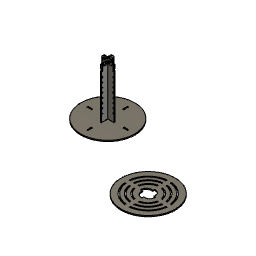
PressurePotRackRotate v5 (Autodesk Fusion 360 design; units mm, degrees)
Autodesk Fusion 360 part; units mm, degrees
(part 1 of 3)
sketch "Sketch1" plane through (0, 0, 0) normal (0, 1, 0) x (1, 0, 0)
  circle A0 centre (0, 0) radius 152.4
  line L0 (0, 0) -> (0, 101.6) construction
  line L1 (0, 0) -> (0, -101.6) construction
  line L2 (0, 0) -> (101.6, 0) construction
  line L3 (0, 0) -> (-101.6, 0) construction
  line L4 (2.9845, 88.9) -> (-2.9845, 88.9)
  line L5 (-2.9845, 88.9) -> (-2.9845, 114.3)
  line L6 (-2.9845, 114.3) -> (2.9845, 114.3)
  line L7 (2.9845, 114.3) -> (2.9845, 88.9)
  line L8 (2.9845, 88.9) -> (-2.9845, 114.3) construction
  line L9 (-2.9845, 88.9) -> (2.9845, 114.3) construction
  line L10 (2.9845, -114.3) -> (-2.9845, -114.3)
  line L11 (-2.9845, -114.3) -> (-2.9845, -88.9)
  line L12 (-2.9845, -88.9) -> (2.9845, -88.9)
  line L13 (2.9845, -88.9) -> (2.9845, -114.3)
  line L14 (2.9845, -114.3) -> (-2.9845, -88.9) construction
  line L15 (-2.9845, -114.3) -> (2.9845, -88.9) construction
  line L16 (114.3, -2.9845) -> (88.9, -2.9845)
  line L17 (88.9, -2.9845) -> (88.9, 2.9845)
  line L18 (88.9, 2.9845) -> (114.3, 2.9845)
  line L19 (114.3, 2.9845) -> (114.3, -2.9845)
  line L20 (114.3, -2.9845) -> (88.9, 2.9845) construction
  line L21 (88.9, -2.9845) -> (114.3, 2.9845) construction
  line L22 (-88.9, -2.9845) -> (-114.3, -2.9845)
  line L23 (-114.3, -2.9845) -> (-114.3, 2.9845)
  line L24 (-114.3, 2.9845) -> (-88.9, 2.9845)
  line L25 (-88.9, 2.9845) -> (-88.9, -2.9845)
  line L26 (-88.9, -2.9845) -> (-114.3, 2.9845) construction
  line L27 (-114.3, -2.9845) -> (-88.9, 2.9845) construction
  line L28 (2.9845, -38.1) -> (-2.9845, -38.1)
  line L29 (-2.9845, -38.1) -> (-2.9845, 38.1)
  line L30 (-2.9845, 38.1) -> (2.9845, 38.1)
  line L31 (2.9845, 38.1) -> (2.9845, -38.1)
  line L32 (2.9845, -38.1) -> (-2.9845, 38.1) construction
  line L33 (-2.9845, -38.1) -> (2.9845, 38.1) construction
  line L34 (38.1, -2.9845) -> (-38.1, -2.9845)
  line L35 (-38.1, -2.9845) -> (-38.1, 2.9845)
  line L36 (-38.1, 2.9845) -> (38.1, 2.9845)
  line L37 (38.1, 2.9845) -> (38.1, -2.9845)
  line L38 (38.1, -2.9845) -> (-38.1, 2.9845) construction
  line L39 (-38.1, -2.9845) -> (38.1, 2.9845) construction
  point P0 (0, 101.6)
  point P1 (0, -101.6)
  point P2 (101.6, 0)
  point P3 (-101.6, 0)
  dimension "d1" = 304.8
  dimension "d2" = 101.6
  dimension "d3" = 101.6
  dimension "d4" = 101.6
  dimension "d5" = 101.6
  dimension "d6" = 5.969
  dimension "d7" = 25.4
  dimension "d8" = 5.969
  dimension "d9" = 25.4
  dimension "d10" = 25.4
  dimension "d11" = 5.969
  dimension "d12" = 25.4
  dimension "d13" = 5.969
  dimension "d14" = 5.969
  dimension "d15" = 76.2
  dimension "d27" = 76.2
  dimension "d28" = 5.969
  constraint coincident A0.centre L0.start
  constraint vertical L0
  constraint parallel L0 L1
  constraint perpendicular L1 L2
  constraint perpendicular L0 L3
  constraint horizontal L4
  constraint perpendicular L4 L5
  constraint parallel L4 L6
  constraint parallel L5 L7
  constraint coincident L8 P0
  constraint coincident L9 P0
  constraint coincident P0 L0.end
  constraint horizontal L10
  constraint perpendicular L10 L11
  constraint parallel L10 L12
  constraint parallel L11 L13
  constraint coincident L14 P1
  constraint coincident L15 P1
  constraint coincident P1 L1.end
  constraint horizontal L16
  constraint perpendicular L16 L17
  constraint parallel L16 L18
  constraint parallel L17 L19
  constraint coincident L20 P2
  constraint coincident L21 P2
  constraint coincident P2 L2.end
  constraint horizontal L22
  constraint perpendicular L22 L23
  constraint parallel L22 L24
  constraint parallel L23 L25
  constraint coincident L26 P3
  constraint coincident L27 P3
  constraint coincident P3 L3.end
  constraint horizontal L28
  constraint perpendicular L28 L29
  constraint parallel L28 L30
  constraint parallel L29 L31
  constraint coincident L32 A0.centre
  constraint coincident L33 A0.centre
  constraint horizontal L34
  constraint perpendicular L34 L35
  constraint parallel L34 L36
  constraint parallel L35 L37
  constraint coincident L38 A0.centre
  constraint coincident L39 A0.centre
  measures "d1" diameter of A0
  measures "d2" distance of A0.centre P0
  measures "d3" distance of A0.centre P1
  measures "d4" distance of A0.centre P2
  measures "d5" distance of A0.centre P3
  measures "d6" distance of L5.end L6.end
  measures "d7" distance of L4.end L5.end
  measures "d8" distance of L11.end L12.end
  measures "d9" distance of L10.end L11.end
  measures "d10" distance of L17.end L18.end
  measures "d11" distance of L16.end L17.end
  measures "d12" distance of L23.end L24.end
  measures "d13" distance of L22.end L23.end
  measures "d14" distance of L29.end L30.end
  measures "d15" distance of L28.end L29.end
  measures "d27" distance of L35.end L36.end
  measures "d28" distance of L34.end L35.end
extrude "Extrude1" add sketch "Sketch1" along normal blind 5.969 contours A0 | L31 L34 L36 L37 | L29 L34 L35 L36 makes body 1 in component "Component"
sketch "Sketch2" plane through (0, 0, 0) normal (0, -1, 0) x (1, 0, 0)
  line L0 (2.9845, 88.9) -> (-2.9845, 88.9)
  line L1 (-2.9845, 88.9) -> (-2.9845, 114.3)
  line L2 (-2.9845, 114.3) -> (2.9845, 114.3)
  line L3 (2.9845, 114.3) -> (2.9845, 88.9)
  line L4 (114.3, -2.9845) -> (88.9, -2.9845)
  line L5 (88.9, -2.9845) -> (88.9, 2.9845)
  line L6 (88.9, 2.9845) -> (114.3, 2.9845)
  line L7 (114.3, 2.9845) -> (114.3, -2.9845)
  line L8 (-88.9, -2.9845) -> (-114.3, -2.9845)
  line L9 (-114.3, -2.9845) -> (-114.3, 2.9845)
  line L10 (-114.3, 2.9845) -> (-88.9, 2.9845)
  line L11 (-88.9, 2.9845) -> (-88.9, -2.9845)
  line L12 (2.9845, -114.3) -> (-2.9845, -114.3)
  line L13 (-2.9845, -114.3) -> (-2.9845, -88.9)
  line L14 (-2.9845, -88.9) -> (2.9845, -88.9)
  line L15 (2.9845, -88.9) -> (2.9845, -114.3)
  line L16 (2.9845, -38.1) -> (-2.9845, -38.1)
  line L17 (-2.9845, -38.1) -> (-2.9845, 38.1)
  line L18 (-2.9845, 38.1) -> (2.9845, 38.1)
  line L19 (2.9845, 38.1) -> (2.9845, -38.1)
  circle A0 centre (0, 0) radius 152.4
  line L20 (-114.3, 2.9845) -> (114.3, 2.9845)
  line L21 (114.3, 2.9845) -> (114.3, -2.9845)
  line L22 (114.3, -2.9845) -> (-114.3, -2.9845)
  line L23 (-114.3, -2.9845) -> (-114.3, 2.9845)
  constraint horizontal L20
  constraint vertical L21
  constraint horizontal L22
  constraint vertical L23
  constraint coincident L4.start L7.end
  constraint coincident L9.end L10.start
extrude "Extrude1'" add sketch "Sketch2" along normal blind 19.05 separate body contours L4 L5 L6 L7 L20 L21 L22 | L5 L19 L20 L22 | L17 L19 L20 L22 | L11 L17 L20 L22 | L8 L9 L10 L11 L20 L22 L23 makes body 2
extrude "Extrude2" add sketch "Sketch2" against normal blind 5.969 contours L4 L5 L6 L7 L20 L21 L22 bodies 2
extrude "Extrude3" add sketch "Sketch2" against normal blind 5.969 contours L8 L9 L10 L11 L20 L22 L23 bodies 2
sketch "Sketch3" plane through (0, -19.05, 0) normal (0, -1, 0) x (1, 0, 0)
  line L0 (-114.3, -2.9845) -> (114.3, -2.9845)
  line L1 (114.3, -2.9845) -> (114.3, 2.9845)
  line L2 (114.3, 2.9845) -> (-114.3, 2.9845)
  line L3 (-114.3, 2.9845) -> (-114.3, -2.9845)
  line L4 (2.9845, -2.9845) -> (-2.9845, -2.9845)
  line L5 (-2.9845, -2.9845) -> (-2.9845, 2.9845)
  line L6 (-2.9845, 2.9845) -> (2.9845, 2.9845)
  line L7 (2.9845, 2.9845) -> (2.9845, -2.9845)
  line L8 (2.9845, -2.9845) -> (-2.9845, 2.9845) construction
  line L9 (-2.9845, -2.9845) -> (2.9845, 2.9845) construction
  dimension "d24" = 5.969
  constraint horizontal L4
  constraint perpendicular L4 L5
  constraint parallel L4 L6
  constraint parallel L5 L7
  constraint coincident L8 origin
  constraint coincident L9 origin
  measures "d24" distance of L5.end L6.end
extrude "Extrude4" cut sketch "Sketch3" against normal blind 9.525 contours L0 L2 L4 L5 L6 L7 bodies 2
copy_body "Body->Comp1" bodies 2 removing the originals makes body 3 in component "Component'"
extrude "Extrude2'" cut sketch "Sketch1" along normal up to surface (5.969 mm away) contours L31 L34 L36 L37 | L29 L34 L35 L36 bodies 1 in component "Component"
sketch "Sketch4" plane through (0, 0, 0) normal (0, -1, 0) x (1, 0, 0)
  line L0 (-38.1, 2.9845) -> (-2.9845, 2.9845)
  line L1 (-2.9845, 2.9845) -> (-2.9845, 38.1)
  line L2 (-2.9845, 38.1) -> (2.9845, 38.1)
  line L3 (2.9845, 38.1) -> (2.9845, 2.9845)
  line L4 (2.9845, 2.9845) -> (38.1, 2.9845)
  line L5 (38.1, 2.9845) -> (38.1, -2.9845)
  line L6 (38.1, -2.9845) -> (2.9845, -2.9845)
  line L7 (2.9845, -2.9845) -> (2.9845, -38.1)
  line L8 (2.9845, -38.1) -> (-2.9845, -38.1)
  line L9 (-2.9845, -38.1) -> (-2.9845, -2.9845)
  line L10 (-2.9845, -2.9845) -> (-38.1, -2.9845)
  line L11 (-38.1, -2.9845) -> (-38.1, 2.9845)
  line L12 (2.9845, -114.3) -> (-2.9845, -114.3)
  line L13 (-2.9845, -114.3) -> (-2.9845, -88.9)
  line L14 (-2.9845, -88.9) -> (2.9845, -88.9)
  line L15 (2.9845, -88.9) -> (2.9845, -114.3)
  line L16 (-88.9, -2.9845) -> (-114.3, -2.9845)
  line L17 (-114.3, -2.9845) -> (-114.3, 2.9845)
  line L18 (-114.3, 2.9845) -> (-88.9, 2.9845)
  line L19 (-88.9, 2.9845) -> (-88.9, -2.9845)
  line L20 (114.3, -2.9845) -> (88.9, -2.9845)
  line L21 (88.9, -2.9845) -> (88.9, 2.9845)
  line L22 (88.9, 2.9845) -> (114.3, 2.9845)
  line L23 (114.3, 2.9845) -> (114.3, -2.9845)
  line L24 (2.9845, 88.9) -> (-2.9845, 88.9)
  line L25 (-2.9845, 88.9) -> (-2.9845, 114.3)
  line L26 (-2.9845, 114.3) -> (2.9845, 114.3)
  line L27 (2.9845, 114.3) -> (2.9845, 88.9)
  circle A0 centre (0, 0) radius 152.4
  line L28 (2.9845, -114.3) -> (-2.9845, -114.3)
  line L29 (-2.9845, -114.3) -> (-2.9845, 114.3)
  line L30 (-2.9845, 114.3) -> (2.9845, 114.3)
  line L31 (2.9845, 114.3) -> (2.9845, -114.3)
  line L32 (2.9845, -114.3) -> (-2.9845, 114.3) construction
  line L33 (-2.9845, -114.3) -> (2.9845, 114.3) construction
  constraint horizontal L28
  constraint perpendicular L28 L29
  constraint parallel L28 L30
  constraint parallel L29 L31
  constraint coincident L12.start L15.end
  constraint coincident L32 A0.centre
  constraint coincident L33 A0.centre
  constraint coincident A0.centre origin
extrude "Extrude1''" add sketch "Sketch4" along normal blind 19.05 separate body contours L1 L2 L3 L7 L8 L9 L29 L31 | L2 L24 L29 L31 | L24 L25 L26 L27 L29 L30 L31 | L8 L14 L29 L31 | L12 L13 L14 L15 L28 L29 L31 makes body 4 in component "Component''"
sketch "Sketch5" plane through (0, 0, 0) normal (0, 1, 0) x (-1, 0, 0)
  line L0 (2.9845, 114.3) -> (-2.9845, 114.3)
  line L1 (-2.9845, 114.3) -> (-2.9845, -114.3)
  line L2 (-2.9845, -114.3) -> (2.9845, -114.3)
  line L3 (2.9845, -114.3) -> (2.9845, 114.3)
  line L4 (-2.9845, 2.9845) -> (2.9845, 2.9845)
  line L5 (2.9845, 2.9845) -> (2.9845, -2.9845)
  line L6 (2.9845, -2.9845) -> (-2.9845, -2.9845)
  line L7 (-2.9845, -2.9845) -> (-2.9845, 2.9845)
  line L8 (-2.9845, 2.9845) -> (2.9845, -2.9845) construction
  line L9 (2.9845, 2.9845) -> (-2.9845, -2.9845) construction
  line L10 (-2.9845, -114.3) -> (2.9845, -114.3)
  line L11 (2.9845, -114.3) -> (2.9845, -88.9)
  line L12 (2.9845, -88.9) -> (-2.9845, -88.9)
  line L13 (-2.9845, -88.9) -> (-2.9845, -114.3)
  line L14 (-2.9845, 114.3) -> (2.9845, 114.3)
  line L15 (2.9845, 114.3) -> (2.9845, 88.9)
  line L16 (2.9845, 88.9) -> (-2.9845, 88.9)
  line L17 (-2.9845, 88.9) -> (-2.9845, 114.3)
  dimension "d33" = 5.969
  dimension "d34" = 25.4
  dimension "d35" = 25.4
  constraint horizontal L4
  constraint perpendicular L4 L5
  constraint parallel L4 L6
  constraint parallel L5 L7
  constraint coincident L8 origin
  constraint coincident L9 origin
  constraint horizontal L10
  constraint vertical L11
  constraint horizontal L12
  constraint vertical L13
  constraint coincident L1.end L2.start
  constraint horizontal L14
  constraint vertical L15
  constraint horizontal L16
  constraint vertical L17
  constraint coincident L0.end L1.start
  measures "d33" distance of L4.end L5.end
  measures "d34" distance of L1.end L12.end
  measures "d35" distance of L0.end L16.end
extrude "Extrude2''" cut sketch "Sketch5" against normal blind 9.525 contours L1 L3 L4 L5 L6 L7 bodies 4 in component "Component''"
extrude "Extrude3'" add sketch "Sketch5" along normal blind 5.969 contours L0 L1 L3 L14 L15 L16 L17 bodies 4 in component "Component''"
extrude "Extrude4'" add sketch "Sketch5" along normal blind 5.969 contours L1 L2 L3 L10 L11 L12 L13 bodies 4 in component "Component''"
sketch "Sketch6" plane through (0, 0, 0) normal (0, 1, 0) x (-1, 0, 0)
  line L0 (88.9, -2.9845) -> (88.9, 2.9845)
  line L1 (88.9, 2.9845) -> (-88.9, 2.9845)
  line L2 (-88.9, 2.9845) -> (-88.9, -2.9845)
  line L3 (-88.9, -2.9845) -> (88.9, -2.9845)
  line L4 (-38.1, 2.9845) -> (38.1, 2.9845)
  line L5 (38.1, 2.9845) -> (38.1, -2.9845)
  line L6 (38.1, -2.9845) -> (-38.1, -2.9845)
  line L7 (-38.1, -2.9845) -> (-38.1, 2.9845)
  line L8 (-38.1, 2.9845) -> (38.1, -2.9845) construction
  line L9 (38.1, 2.9845) -> (-38.1, -2.9845) construction
  dimension "d42" = 76.2
  constraint horizontal L4
  constraint perpendicular L4 L5
  constraint parallel L4 L6
  constraint parallel L5 L7
  constraint coincident L8 origin
  constraint coincident L9 origin
  measures "d42" distance of L5.end L6.end
extrude "Extrude1'''" add sketch "Sketch6" along normal blind 304.8 contours L1 L3 L4 L5 L6 L7 bodies 3 in component "Component'"
sketch "Sketch7" plane through (0, 0, 0) normal (0, 1, 0) x (-1, 0, 0)
  line L0 (2.9845, 88.9) -> (-2.9845, 88.9)
  line L1 (-2.9845, 88.9) -> (-2.9845, 2.9845)
  line L2 (-2.9845, 2.9845) -> (2.9845, 2.9845)
  line L3 (2.9845, 2.9845) -> (2.9845, 88.9)
  line L4 (2.9845, 2.9845) -> (-2.9845, 2.9845)
  line L5 (-2.9845, 2.9845) -> (-2.9845, 38.1)
  line L6 (-2.9845, 38.1) -> (2.9845, 38.1)
  line L7 (2.9845, 38.1) -> (2.9845, 2.9845)
  dimension "d45" = 35.1155
  constraint horizontal L4
  constraint vertical L5
  constraint horizontal L6
  constraint vertical L7
  constraint coincident L2.end L3.start
  measures "d45" distance of L2.end L6.end
extrude "Extrude5" add sketch "Sketch7" along normal blind 304.8 contours L1 L2 L3 L4 L5 L6 L7 bodies 4 in component "Component''"
sketch "Sketch8" plane through (0, 0, 0) normal (0, 1, 0) x (-1, 0, 0)
  line L0 (-2.9845, -88.9) -> (2.9845, -88.9)
  line L1 (2.9845, -88.9) -> (2.9845, -2.9845)
  line L2 (2.9845, -2.9845) -> (-2.9845, -2.9845)
  line L3 (-2.9845, -2.9845) -> (-2.9845, -88.9)
  line L4 (2.9845, -2.9845) -> (-2.9845, -2.9845)
  line L5 (-2.9845, -2.9845) -> (-2.9845, -38.1)
  line L6 (-2.9845, -38.1) -> (2.9845, -38.1)
  line L7 (2.9845, -38.1) -> (2.9845, -2.9845)
  dimension "d48" = 35.1155
  constraint horizontal L4
  constraint vertical L5
  constraint horizontal L6
  constraint vertical L7
  constraint coincident L1.end L2.start
  measures "d48" distance of L1.end L6.end
extrude "Extrude6" add sketch "Sketch8" along normal blind 304.8 contours L1 L2 L3 L4 L5 L6 L7 bodies 4 in component "Component''"
fillet "Fillet1" radius 12.7 2 edges at (114.3, -19.05, 0) (-114.3, -19.05, 0) on bodies 3 in component "Component'"
fillet "Fillet1'" radius 12.7 2 edges at (0, -19.05, 114.3) (0, -19.05, -114.3) on bodies 4 in component "Component''"
sketch "Sketch9" plane through (-38.1, 0, 0) normal (-1, 0, 0) x (0, 0, 1)
  line L0 (-2.9845, 0) -> (2.9845, 0)
  line L1 (2.9845, 0) -> (2.9845, 304.8)
  line L2 (2.9845, 304.8) -> (-2.9845, 304.8)
  line L3 (-2.9845, 304.8) -> (-2.9845, 0)
  line L4 (-2.9845, 304.8) -> (2.9845, 304.8)
  line L5 (2.9845, 304.8) -> (2.9845, 254)
  line L6 (2.9845, 254) -> (-2.9845, 254)
  line L7 (-2.9845, 254) -> (-2.9845, 304.8)
  dimension "d55" = 50.8
  constraint horizontal L4
  constraint vertical L5
  constraint horizontal L6
  constraint vertical L7
  constraint coincident L2.end L3.start
  measures "d55" distance of L2.end L6.end
extrude "Extrude2'''" cut sketch "Sketch9" against normal blind 6.35 contours L1 L2 L3 L4 L5 L6 L7 bodies 3 in component "Component'"
sketch "Sketch10" plane through (0, 0, -38.1) normal (0, 0, -1) x (-1, 0, 0)
  line L0 (-2.9845, 0) -> (2.9845, 0)
  line L1 (2.9845, 0) -> (2.9845, 304.8)
  line L2 (2.9845, 304.8) -> (-2.9845, 304.8)
  line L3 (-2.9845, 304.8) -> (-2.9845, 0)
  line L4 (-2.9845, 304.8) -> (2.9845, 304.8)
  line L5 (2.9845, 304.8) -> (2.9845, 254)
  line L6 (2.9845, 254) -> (-2.9845, 254)
  line L7 (-2.9845, 254) -> (-2.9845, 304.8)
  dimension "d58" = 50.8
  constraint horizontal L4
  constraint vertical L5
  constraint horizontal L6
  constraint vertical L7
  constraint coincident L2.end L3.start
  measures "d58" distance of L2.end L6.end
extrude "Extrude7" cut sketch "Sketch10" against normal blind 6.35 contours L1 L2 L3 L4 L5 L6 L7 bodies 4 in component "Component''"
sketch "Sketch11" plane through (38.1, 0, 0) normal (1, 0, 0) x (0, 0, -1)
  line L0 (-2.9845, 0) -> (2.9845, 0)
  line L1 (2.9845, 0) -> (2.9845, 304.8)
  line L2 (2.9845, 304.8) -> (-2.9845, 304.8)
  line L3 (-2.9845, 304.8) -> (-2.9845, 0)
  line L4 (-2.9845, 304.8) -> (2.9845, 304.8)
  line L5 (2.9845, 304.8) -> (2.9845, 254)
  line L6 (2.9845, 254) -> (-2.9845, 254)
  line L7 (-2.9845, 254) -> (-2.9845, 304.8)
  dimension "d61" = 5.969
  dimension "d62" = 50.8
  constraint horizontal L4
  constraint vertical L5
  constraint horizontal L6
  constraint vertical L7
  constraint coincident L2.end L3.start
  measures "d61" distance of L2.end L1.end
  measures "d62" distance of L2.end L6.end
extrude "Extrude3''" cut sketch "Sketch11" against normal blind 6.35 contours L1 L2 L3 L4 L5 L6 L7 bodies 3 in component "Component'"
sketch "Sketch12" plane through (0, 0, 38.1) normal (0, 0, 1) x (1, 0, 0)
  line L0 (-2.9845, 0) -> (2.9845, 0)
  line L1 (2.9845, 0) -> (2.9845, 304.8)
  line L2 (2.9845, 304.8) -> (-2.9845, 304.8)
  line L3 (-2.9845, 304.8) -> (-2.9845, 0)
  line L4 (-2.9845, 304.8) -> (2.9845, 304.8)
  line L5 (2.9845, 304.8) -> (2.9845, 254)
  line L6 (2.9845, 254) -> (-2.9845, 254)
  line L7 (-2.9845, 254) -> (-2.9845, 304.8)
  dimension "d65" = 50.8
  constraint horizontal L4
  constraint vertical L5
  constraint horizontal L6
  constraint vertical L7
  constraint coincident L2.end L3.start
  measures "d65" distance of L2.end L6.end
extrude "Extrude8" cut sketch "Sketch12" against normal blind 6.35 contours L1 L2 L3 L4 L5 L6 L7 bodies 4 in component "Component''"
fillet "Fillet2" radius 12.7 2 edges at (31.75, 304.8, 0) (-31.75, 304.8, 0) on bodies 3 in component "Component'"
fillet "Fillet2'" radius 12.7 2 edges at (0, 304.8, -31.75) (0, 304.8, 31.75) on bodies 4 in component "Component''"
sketch "Sketch13" plane through (-2.9845, 0, 0) normal (-1, 0, 0) x (0, 0, 1)
  arc A0 (31.75, 292.1) -> (19.05, 304.8) centre (19.05, 292.1) ccw
  line L0 (19.05, 304.8) -> (2.9845, 304.8)
  line L1 (2.9845, 304.8) -> (2.9845, -9.525)
  line L2 (2.9845, -9.525) -> (-2.9845, -9.525)
  line L3 (-2.9845, -9.525) -> (-2.9845, 304.8)
  line L4 (-2.9845, 304.8) -> (-19.05, 304.8)
  arc A1 (-19.05, 304.8) -> (-31.75, 292.1) centre (-19.05, 292.1) ccw
  line L5 (-31.75, 292.1) -> (-31.75, 254)
  line L6 (-31.75, 254) -> (-38.1, 254)
  line L7 (-38.1, 254) -> (-38.1, 0)
  line L8 (-38.1, 0) -> (-88.9, 0)
  line L9 (-88.9, 0) -> (-88.9, 5.969)
  line L10 (-88.9, 5.969) -> (-114.3, 5.969)
  line L11 (-114.3, 5.969) -> (-114.3, -6.35)
  arc A2 (-114.3, -6.35) -> (-101.6, -19.05) centre (-101.6, -6.35) ccw
  line L12 (-101.6, -19.05) -> (101.6, -19.05)
  arc A3 (101.6, -19.05) -> (114.3, -6.35) centre (101.6, -6.35) ccw
  line L13 (114.3, -6.35) -> (114.3, 5.969)
  line L14 (114.3, 5.969) -> (88.9, 5.969)
  line L15 (88.9, 5.969) -> (88.9, 0)
  line L16 (88.9, 0) -> (38.1, 0)
  line L17 (38.1, 0) -> (38.1, 254)
  line L18 (38.1, 254) -> (31.75, 254)
  line L19 (31.75, 254) -> (31.75, 292.1)
  line L20 (2.9845, 304.8) -> (17.3736, 304.8) construction
  line L21 (17.3736, 304.8) -> (17.3736, 285.75) construction
  line L22 (-2.9845, 304.8) -> (-17.3736, 304.8) construction
  line L23 (-17.3736, 304.8) -> (-17.3736, 285.75) construction
  circle A4 centre (17.3736, 285.75) radius 11.1125
  circle A5 centre (-17.3736, 285.75) radius 11.1125
  dimension "d72" = 14.3891
  dimension "d73" = 19.05
  dimension "d74" = 14.3891
  dimension "d75" = 19.05
  dimension "d76" = 22.225
  dimension "d77" = 22.225
  constraint coincident L0.end L1.start
  constraint perpendicular L1 L20
  constraint perpendicular L20 L21
  constraint coincident L3.end L4.start
  constraint perpendicular L3 L22
  constraint perpendicular L22 L23
  constraint coincident L21.end A4.centre
  constraint coincident L23.end A5.centre
  measures "d72" distance of L0.end L20.end
  measures "d73" distance of L20.end L21.end
  measures "d74" distance of L3.end L22.end
  measures "d75" distance of L22.end L23.end
  measures "d76" diameter of A4
  measures "d77" diameter of A5
extrude "Extrude9" cut sketch "Sketch13" against normal up to surface (5.969 mm away) contours A4 bodies 4 in component "Component''"
extrude "Extrude10" cut sketch "Sketch13" against normal up to surface (5.969 mm away) contours A5 bodies 4 in component "Component''"
sketch "Sketch14" plane through (0, 0, -2.9845) normal (0, 0, -1) x (-1, 0, 0)
  arc A0 (31.75, 292.1) -> (19.05, 304.8) centre (19.05, 292.1) ccw
  line L0 (19.05, 304.8) -> (-19.05, 304.8)
  arc A1 (-19.05, 304.8) -> (-31.75, 292.1) centre (-19.05, 292.1) ccw
  line L1 (-31.75, 292.1) -> (-31.75, 254)
  line L2 (-31.75, 254) -> (-38.1, 254)
  line L3 (-38.1, 254) -> (-38.1, 0)
  line L4 (-38.1, 0) -> (-88.9, 0)
  line L5 (-88.9, 0) -> (-88.9, 5.969)
  line L6 (-88.9, 5.969) -> (-114.3, 5.969)
  line L7 (-114.3, 5.969) -> (-114.3, -6.35)
  arc A2 (-114.3, -6.35) -> (-101.6, -19.05) centre (-101.6, -6.35) ccw
  line L8 (-101.6, -19.05) -> (-2.9845, -19.05)
  line L9 (-2.9845, -19.05) -> (-2.9845, -9.525)
  line L10 (-2.9845, -9.525) -> (2.9845, -9.525)
  line L11 (2.9845, -9.525) -> (2.9845, -19.05)
  line L12 (2.9845, -19.05) -> (101.6, -19.05)
  arc A3 (101.6, -19.05) -> (114.3, -6.35) centre (101.6, -6.35) ccw
  line L13 (114.3, -6.35) -> (114.3, 5.969)
  line L14 (114.3, 5.969) -> (88.9, 5.969)
  line L15 (88.9, 5.969) -> (88.9, 0)
  line L16 (88.9, 0) -> (38.1, 0)
  line L17 (38.1, 0) -> (38.1, 254)
  line L18 (38.1, 254) -> (31.75, 254)
  line L19 (31.75, 254) -> (31.75, 292.1)
  line L20 (-31.75, 292.1) -> (-31.75, 285.75) construction
  line L21 (31.75, 292.1) -> (31.75, 285.75) construction
  line L22 (-31.75, 285.75) -> (-17.3609, 285.75) construction
  line L23 (31.75, 285.75) -> (17.3609, 285.75) construction
  circle A4 centre (17.3609, 285.75) radius 11.1125
  circle A5 centre (-17.3609, 285.75) radius 11.1125
  dimension "d82" = 6.35
  dimension "d83" = 6.35
  dimension "d84" = 14.3891
  dimension "d85" = 14.3891
  dimension "d86" = 22.225
  dimension "d87" = 22.225
  constraint coincident A1.end L1.start
  constraint perpendicular L0 L20
  constraint coincident A0.start L19.end
  constraint parallel L19 L21
  constraint perpendicular L20 L22
  constraint perpendicular L21 L23
  constraint coincident L23.end A4.centre
  constraint coincident L22.end A5.centre
  measures "d82" distance of A1.end L20.end
  measures "d83" distance of A0.start L21.end
  measures "d84" distance of L20.end L22.end
  measures "d85" distance of L21.end L23.end
  measures "d86" diameter of A4
  measures "d87" diameter of A5
extrude "Extrude4''" cut sketch "Sketch14" against normal up to surface (5.969 mm away) contours A4 | A5 bodies 3 in component "Component'"
sketch "Sketch15" plane through (0, 0, 0) normal (0, 1, 0) x (1, 0, 0)
  circle A0 centre (482.6, -254) radius 152.4
  line L0 (485.5845, -285.75) -> (479.6155, -285.75)
  line L1 (479.6155, -285.75) -> (479.6155, -222.25)
  line L2 (479.6155, -222.25) -> (485.5845, -222.25)
  line L3 (485.5845, -222.25) -> (485.5845, -285.75)
  line L4 (485.5845, -285.75) -> (479.6155, -222.25) construction
  line L5 (479.6155, -285.75) -> (485.5845, -222.25) construction
  line L6 (514.35, -256.9845) -> (450.85, -256.9845)
  line L7 (450.85, -256.9845) -> (450.85, -251.0155)
  line L8 (450.85, -251.0155) -> (514.35, -251.0155)
  line L9 (514.35, -251.0155) -> (514.35, -256.9845)
  line L10 (514.35, -256.9845) -> (450.85, -251.0155) construction
  line L11 (450.85, -256.9845) -> (514.35, -251.0155) construction
  point P0 (482.6, -254)
  point P1 (482.6, -254)
  dimension "d90" = 304.8
  dimension "d91" = 5.969
  dimension "d92" = 63.5
  dimension "d93" = 63.5
  dimension "d94" = 5.969
  constraint horizontal L0
  constraint perpendicular L0 L1
  constraint parallel L0 L2
  constraint parallel L1 L3
  constraint coincident L4 P1
  constraint coincident L5 P1
  constraint coincident P0 A0.centre
  constraint horizontal L6
  constraint perpendicular L6 L7
  constraint parallel L6 L8
  constraint parallel L7 L9
  constraint coincident L10 P1
  constraint coincident L11 P1
  constraint coincident P1 P0
  measures "d90" diameter of A0
  measures "d91" distance of L1.end L2.end
  measures "d92" distance of L0.end L1.end
  measures "d93" distance of L7.end L8.end
  measures "d94" distance of L6.end L7.end
extrude "Extrude5'" add sketch "Sketch15" along normal blind 5.969 separate body makes body 5
sketch "Sketch16" plane through (0, 5.969, 0) normal (0, 1, 0) x (-1, 0, 0)
  line L0 (-485.5845, 251.0155) -> (-514.35, 251.0155)
  line L1 (-514.35, 251.0155) -> (-514.35, 256.9845)
  line L2 (-514.35, 256.9845) -> (-485.5845, 256.9845)
  line L3 (-485.5845, 256.9845) -> (-485.5845, 285.75)
  line L4 (-485.5845, 285.75) -> (-479.6155, 285.75)
  line L5 (-479.6155, 285.75) -> (-479.6155, 256.9845)
  line L6 (-479.6155, 256.9845) -> (-450.85, 256.9845)
  line L7 (-450.85, 256.9845) -> (-450.85, 251.0155)
  line L8 (-450.85, 251.0155) -> (-479.6155, 251.0155)
  line L9 (-479.6155, 251.0155) -> (-479.6155, 222.25)
  line L10 (-479.6155, 222.25) -> (-485.5845, 222.25)
  line L11 (-485.5845, 222.25) -> (-485.5845, 251.0155)
  circle A0 centre (-482.6, 254) radius 152.4
  circle A1 centre (-482.6, 254) radius 63.5
  circle A2 centre (-482.6, 254) radius 69.85
  circle A3 centre (-482.6, 254) radius 88.9
  circle A4 centre (-482.6, 254) radius 95.25
  circle A5 centre (-482.6, 254) radius 114.3
  circle A6 centre (-482.6, 254) radius 120.65
  line L12 (-495.3, 381) -> (-469.9, 381)
  line L13 (-469.9, 381) -> (-469.9, 127)
  line L14 (-469.9, 127) -> (-495.3, 127)
  line L15 (-495.3, 127) -> (-495.3, 381)
  line L16 (-495.3, 381) -> (-469.9, 127) construction
  line L17 (-469.9, 381) -> (-495.3, 127) construction
  line L18 (-609.6, 266.7) -> (-355.6, 266.7)
  line L19 (-355.6, 266.7) -> (-355.6, 241.3)
  line L20 (-355.6, 241.3) -> (-609.6, 241.3)
  line L21 (-609.6, 241.3) -> (-609.6, 266.7)
  line L22 (-609.6, 266.7) -> (-355.6, 241.3) construction
  line L23 (-355.6, 266.7) -> (-609.6, 241.3) construction
  point P0 (-482.6, 254)
  point P1 (-482.6, 254)
  dimension "d98" = 127
  dimension "d99" = 139.7
  dimension "d100" = 177.8
  dimension "d101" = 190.5
  dimension "d102" = 228.6
  dimension "d103" = 241.3
  dimension "d104" = 254
  dimension "d105" = 25.4
  constraint concentric A0 A1
  constraint concentric A1 A2
  constraint concentric A2 A3
  constraint concentric A1 A4
  constraint concentric A3 A5
  constraint concentric A3 A6
  constraint horizontal L12
  constraint perpendicular L12 L13
  constraint parallel L12 L14
  constraint parallel L13 L15
  constraint coincident L16 P1
  constraint coincident L17 P1
  constraint coincident P1 P0
  constraint horizontal L18
  constraint perpendicular L18 L19
  constraint parallel L18 L20
  constraint parallel L19 L21
  constraint coincident L22 P1
  constraint coincident L23 P1
  measures "d98" diameter of A1
  measures "d99" diameter of A2
  measures "d100" diameter of A3
  measures "d101" diameter of A4
  measures "d102" diameter of A5
  measures "d103" diameter of A6
  measures "d104" distance of L19.end L20.end
  measures "d105" distance of L18.end L19.end
extrude "Extrude6'" cut sketch "Sketch16" against normal up to surface (5.969 mm away) contours A1 A2 L15 L20 | A1 A2 L13 L20 | A1 A2 L15 L18 | A3 A4 L15 L20 | A1 A2 L13 L18 | A3 A4 L13 L20 | A3 A4 L15 L18 | A5 A6 L15 L20 | A3 A4 L13 L18 | A5 A6 L13 L20 | A5 A6 L15 L18 | A5 A6 L13 L18 bodies 5
copy_body "Body->Comp2" bodies 5 removing the originals makes body 6 in component "Component'''"
sketch "Sketch17" plane through (0, 5.969, 0) normal (0, 1, 0) x (-1, 0, 0)
  arc A0 (-495.3, 367.5922) -> (-596.1922, 266.7) centre (-482.6, 254) ccw
  line L0 (-596.1922, 266.7) -> (-602.5797, 266.7)
  arc A1 (-495.3, 373.9797) -> (-602.5797, 266.7) centre (-482.6, 254) ccw
  line L1 (-495.3, 373.9797) -> (-495.3, 367.5922)
  arc A2 (-469.9, 166.0118) -> (-394.6118, 241.3) centre (-482.6, 254) ccw
  line L2 (-394.6118, 241.3) -> (-388.2005, 241.3)
  arc A3 (-469.9, 159.6005) -> (-388.2005, 241.3) centre (-482.6, 254) ccw
  line L3 (-469.9, 159.6005) -> (-469.9, 166.0118)
  arc A4 (-420.383, 266.7) -> (-469.9, 316.217) centre (-482.6, 254) ccw
  line L4 (-469.9, 316.217) -> (-469.9, 322.6857)
  arc A5 (-413.9142, 266.7) -> (-469.9, 322.6857) centre (-482.6, 254) ccw
  line L5 (-413.9142, 266.7) -> (-420.383, 266.7)
  arc A6 (-469.9, 191.783) -> (-420.383, 241.3) centre (-482.6, 254) ccw
  line L6 (-420.383, 241.3) -> (-413.9142, 241.3)
  arc A7 (-469.9, 185.3142) -> (-413.9142, 241.3) centre (-482.6, 254) ccw
  line L7 (-469.9, 185.3142) -> (-469.9, 191.783)
  arc A8 (-394.6118, 266.7) -> (-469.9, 341.9882) centre (-482.6, 254) ccw
  line L8 (-469.9, 341.9882) -> (-469.9, 348.3995)
  arc A9 (-388.2005, 266.7) -> (-469.9, 348.3995) centre (-482.6, 254) ccw
  line L9 (-388.2005, 266.7) -> (-394.6118, 266.7)
  arc A10 (-469.9, 140.4077) -> (-369.0077, 241.3) centre (-482.6, 254) ccw
  line L10 (-369.0077, 241.3) -> (-362.6203, 241.3)
  arc A11 (-469.9, 134.0203) -> (-362.6203, 241.3) centre (-482.6, 254) ccw
  line L11 (-469.9, 134.0203) -> (-469.9, 140.4077)
  arc A12 (-369.0077, 266.7) -> (-469.9, 367.5922) centre (-482.6, 254) ccw
  line L12 (-469.9, 367.5922) -> (-469.9, 373.9797)
  arc A13 (-362.6203, 266.7) -> (-469.9, 373.9797) centre (-482.6, 254) ccw
  line L13 (-362.6203, 266.7) -> (-369.0077, 266.7)
  arc A14 (-570.5882, 241.3) -> (-495.3, 166.0118) centre (-482.6, 254) ccw
  line L14 (-495.3, 166.0118) -> (-495.3, 159.6005)
  arc A15 (-576.9995, 241.3) -> (-495.3, 159.6005) centre (-482.6, 254) ccw
  line L15 (-576.9995, 241.3) -> (-570.5882, 241.3)
  arc A16 (-495.3, 316.217) -> (-544.817, 266.7) centre (-482.6, 254) ccw
  line L16 (-544.817, 266.7) -> (-551.2857, 266.7)
  arc A17 (-495.3, 322.6857) -> (-551.2857, 266.7) centre (-482.6, 254) ccw
  line L17 (-495.3, 322.6857) -> (-495.3, 316.217)
  arc A18 (-544.817, 241.3) -> (-495.3, 191.783) centre (-482.6, 254) ccw
  line L18 (-495.3, 191.783) -> (-495.3, 185.3142)
  arc A19 (-551.2857, 241.3) -> (-495.3, 185.3142) centre (-482.6, 254) ccw
  line L19 (-551.2857, 241.3) -> (-544.817, 241.3)
  arc A20 (-495.3, 341.9882) -> (-570.5882, 266.7) centre (-482.6, 254) ccw
  line L20 (-570.5882, 266.7) -> (-576.9995, 266.7)
  arc A21 (-495.3, 348.3995) -> (-576.9995, 266.7) centre (-482.6, 254) ccw
  line L21 (-495.3, 348.3995) -> (-495.3, 341.9882)
  arc A22 (-596.1922, 241.3) -> (-495.3, 140.4077) centre (-482.6, 254) ccw
  line L22 (-495.3, 140.4077) -> (-495.3, 134.0203)
  arc A23 (-602.5797, 241.3) -> (-495.3, 134.0203) centre (-482.6, 254) ccw
  line L23 (-602.5797, 241.3) -> (-596.1922, 241.3)
  line L24 (-485.5845, 251.0155) -> (-514.35, 251.0155)
  line L25 (-514.35, 251.0155) -> (-514.35, 256.9845)
  line L26 (-514.35, 256.9845) -> (-485.5845, 256.9845)
  line L27 (-485.5845, 256.9845) -> (-485.5845, 285.75)
  line L28 (-485.5845, 285.75) -> (-479.6155, 285.75)
  line L29 (-479.6155, 285.75) -> (-479.6155, 256.9845)
  line L30 (-479.6155, 256.9845) -> (-450.85, 256.9845)
  line L31 (-450.85, 256.9845) -> (-450.85, 251.0155)
  line L32 (-450.85, 251.0155) -> (-479.6155, 251.0155)
  line L33 (-479.6155, 251.0155) -> (-479.6155, 222.25)
  line L34 (-479.6155, 222.25) -> (-485.5845, 222.25)
  line L35 (-485.5845, 222.25) -> (-485.5845, 251.0155)
  circle A24 centre (-482.6, 254) radius 152.4
sketch "Sketch18" plane through (0, 5.969, 0) normal (0, 1, 0) x (-1, 0, 0)
  circle A0 centre (0, 0) radius 152.4
  line L0 (2.9845, 88.9) -> (-2.9845, 88.9)
  line L1 (-2.9845, 88.9) -> (-2.9845, 114.3)
  line L2 (-2.9845, 114.3) -> (2.9845, 114.3)
  line L3 (2.9845, 114.3) -> (2.9845, 88.9)
  line L4 (-88.9, -2.9845) -> (-114.3, -2.9845)
  line L5 (-114.3, -2.9845) -> (-114.3, 2.9845)
  line L6 (-114.3, 2.9845) -> (-88.9, 2.9845)
  line L7 (-88.9, 2.9845) -> (-88.9, -2.9845)
  line L8 (2.9845, 2.9845) -> (38.1, 2.9845)
  line L9 (38.1, 2.9845) -> (38.1, -2.9845)
  line L10 (38.1, -2.9845) -> (2.9845, -2.9845)
  line L11 (2.9845, -2.9845) -> (2.9845, -38.1)
  line L12 (2.9845, -38.1) -> (-2.9845, -38.1)
  line L13 (-2.9845, -38.1) -> (-2.9845, -2.9845)
  line L14 (-2.9845, -2.9845) -> (-38.1, -2.9845)
  line L15 (-38.1, -2.9845) -> (-38.1, 2.9845)
  line L16 (-38.1, 2.9845) -> (-2.9845, 2.9845)
  line L17 (-2.9845, 2.9845) -> (-2.9845, 38.1)
  line L18 (-2.9845, 38.1) -> (2.9845, 38.1)
  line L19 (2.9845, 38.1) -> (2.9845, 2.9845)
  line L20 (114.3, -2.9845) -> (88.9, -2.9845)
  line L21 (88.9, -2.9845) -> (88.9, 2.9845)
  line L22 (88.9, 2.9845) -> (114.3, 2.9845)
  line L23 (114.3, 2.9845) -> (114.3, -2.9845)
  line L24 (2.9845, -114.3) -> (-2.9845, -114.3)
  line L25 (-2.9845, -114.3) -> (-2.9845, -88.9)
  line L26 (-2.9845, -88.9) -> (2.9845, -88.9)
  line L27 (2.9845, -88.9) -> (2.9845, -114.3)
sketch "Sketch21" plane through (-2.9845, 0, 0) normal (-1, 0, 0) x (0, 0, 1)
  circle A0 centre (-17.3736, 285.75) radius 11.1125
  circle A1 centre (17.3736, 285.75) radius 11.1125
  arc A2 (31.75, 292.1) -> (19.05, 304.8) centre (19.05, 292.1) ccw
  line L0 (19.05, 304.8) -> (2.9845, 304.8)
  line L1 (2.9845, 304.8) -> (2.9845, -9.525)
  line L2 (2.9845, -9.525) -> (-2.9845, -9.525)
  line L3 (-2.9845, -9.525) -> (-2.9845, 304.8)
  line L4 (-2.9845, 304.8) -> (-19.05, 304.8)
  arc A3 (-19.05, 304.8) -> (-31.75, 292.1) centre (-19.05, 292.1) ccw
  line L5 (-31.75, 292.1) -> (-31.75, 254)
  line L6 (-31.75, 254) -> (-38.1, 254)
  line L7 (-38.1, 254) -> (-38.1, 0)
  line L8 (-38.1, 0) -> (-88.9, 0)
  line L9 (-88.9, 0) -> (-88.9, 5.969)
  line L10 (-88.9, 5.969) -> (-114.3, 5.969)
  line L11 (-114.3, 5.969) -> (-114.3, -6.35)
  arc A4 (-114.3, -6.35) -> (-101.6, -19.05) centre (-101.6, -6.35) ccw
  line L12 (-101.6, -19.05) -> (101.6, -19.05)
  arc A5 (101.6, -19.05) -> (114.3, -6.35) centre (101.6, -6.35) ccw
  line L13 (114.3, -6.35) -> (114.3, 5.969)
  line L14 (114.3, 5.969) -> (88.9, 5.969)
  line L15 (88.9, 5.969) -> (88.9, 0)
  line L16 (88.9, 0) -> (38.1, 0)
  line L17 (38.1, 0) -> (38.1, 254)
  line L18 (38.1, 254) -> (31.75, 254)
  line L19 (31.75, 254) -> (31.75, 292.1)
sketch "Sketch22" plane through (0, 0, 2.9845) normal (0, 0, 1) x (1, 0, 0)
  circle A0 centre (17.3609, 285.75) radius 11.1125
  circle A1 centre (-17.3609, 285.75) radius 11.1125
  arc A2 (-19.05, 304.8) -> (-31.75, 292.1) centre (-19.05, 292.1) ccw
  line L0 (-31.75, 292.1) -> (-31.75, 254)
  line L1 (-31.75, 254) -> (-38.1, 254)
  line L2 (-38.1, 254) -> (-38.1, 0)
  line L3 (-38.1, 0) -> (-88.9, 0)
  line L4 (-88.9, 0) -> (-88.9, 5.969)
  line L5 (-88.9, 5.969) -> (-114.3, 5.969)
  line L6 (-114.3, 5.969) -> (-114.3, -6.35)
  arc A3 (-114.3, -6.35) -> (-101.6, -19.05) centre (-101.6, -6.35) ccw
  line L7 (-101.6, -19.05) -> (-2.9845, -19.05)
  line L8 (-2.9845, -19.05) -> (-2.9845, -9.525)
  line L9 (-2.9845, -9.525) -> (2.9845, -9.525)
  line L10 (2.9845, -9.525) -> (2.9845, -19.05)
  line L11 (2.9845, -19.05) -> (101.6, -19.05)
  arc A4 (101.6, -19.05) -> (114.3, -6.35) centre (101.6, -6.35) ccw
  line L12 (114.3, -6.35) -> (114.3, 5.969)
  line L13 (114.3, 5.969) -> (88.9, 5.969)
  line L14 (88.9, 5.969) -> (88.9, 0)
  line L15 (88.9, 0) -> (38.1, 0)
  line L16 (38.1, 0) -> (38.1, 254)
  line L17 (38.1, 254) -> (31.75, 254)
  line L18 (31.75, 254) -> (31.75, 292.1)
  arc A5 (31.75, 292.1) -> (19.05, 304.8) centre (19.05, 292.1) ccw
  line L19 (19.05, 304.8) -> (-19.05, 304.8)
sketch "Sketch23" plane through (0, 0, -2.9845) normal (0, 0, -1) x (-1, 0, 0)
  circle A0 centre (-17.3609, 285.75) radius 11.1125
  circle A1 centre (17.3609, 285.75) radius 11.1125
  arc A2 (31.75, 292.1) -> (19.05, 304.8) centre (19.05, 292.1) ccw
  line L0 (19.05, 304.8) -> (-19.05, 304.8)
  arc A3 (-19.05, 304.8) -> (-31.75, 292.1) centre (-19.05, 292.1) ccw
  line L1 (-31.75, 292.1) -> (-31.75, 254)
  line L2 (-31.75, 254) -> (-38.1, 254)
  line L3 (-38.1, 254) -> (-38.1, 0)
  line L4 (-38.1, 0) -> (-88.9, 0)
  line L5 (-88.9, 0) -> (-88.9, 5.969)
  line L6 (-88.9, 5.969) -> (-114.3, 5.969)
  line L7 (-114.3, 5.969) -> (-114.3, -6.35)
  arc A4 (-114.3, -6.35) -> (-101.6, -19.05) centre (-101.6, -6.35) ccw
  line L8 (-101.6, -19.05) -> (-2.9845, -19.05)
  line L9 (-2.9845, -19.05) -> (-2.9845, -9.525)
  line L10 (-2.9845, -9.525) -> (2.9845, -9.525)
  line L11 (2.9845, -9.525) -> (2.9845, -19.05)
  line L12 (2.9845, -19.05) -> (101.6, -19.05)
  arc A5 (101.6, -19.05) -> (114.3, -6.35) centre (101.6, -6.35) ccw
  line L13 (114.3, -6.35) -> (114.3, 5.969)
  line L14 (114.3, 5.969) -> (88.9, 5.969)
  line L15 (88.9, 5.969) -> (88.9, 0)
  line L16 (88.9, 0) -> (38.1, 0)
  line L17 (38.1, 0) -> (38.1, 254)
  line L18 (38.1, 254) -> (31.75, 254)
  line L19 (31.75, 254) -> (31.75, 292.1)
  line L20 (0, 304.8) -> (0, 228.6) construction
  line L21 (0, 228.6) -> (2.9845, 228.6) construction
  line L22 (0, 228.6) -> (-2.9845, 228.6) construction
  line L23 (2.9845, 228.6) -> (15.6845, 228.6)
  line L24 (15.6845, 228.6) -> (15.6845, 222.631)
  line L25 (15.6845, 222.631) -> (2.9845, 222.631)
  line L26 (2.9845, 222.631) -> (2.9845, 228.6)
  line L27 (-2.9845, 228.6) -> (-15.6845, 228.6)
  line L28 (-15.6845, 228.6) -> (-15.6845, 222.631)
  line L29 (-15.6845, 222.631) -> (-2.9845, 222.631)
  line L30 (-2.9845, 222.631) -> (-2.9845, 228.6)
  line L31 (2.9845, 228.6) -> (2.9845, 177.8) construction
  line L32 (-2.9845, 228.6) -> (-2.9845, 177.8) construction
  line L33 (2.9845, 177.8) -> (15.6845, 177.8)
  line L34 (15.6845, 177.8) -> (15.6845, 171.831)
  line L35 (15.6845, 171.831) -> (2.9845, 171.831)
  line L36 (2.9845, 171.831) -> (2.9845, 177.8)
  line L37 (-2.9845, 177.8) -> (-15.6845, 177.8)
  line L38 (-15.6845, 177.8) -> (-15.6845, 171.831)
  line L39 (-15.6845, 171.831) -> (-2.9845, 171.831)
  line L40 (-2.9845, 171.831) -> (-2.9845, 177.8)
  line L41 (2.9845, 177.8) -> (2.9845, 127) construction
  line L42 (-2.9845, 177.8) -> (-2.9845, 127) construction
  line L43 (2.9845, 127) -> (15.6845, 127)
  line L44 (15.6845, 127) -> (15.6845, 121.031)
  line L45 (15.6845, 121.031) -> (2.9845, 121.031)
  line L46 (2.9845, 121.031) -> (2.9845, 127)
  line L47 (-2.9845, 127) -> (-15.6845, 127)
  line L48 (-15.6845, 127) -> (-15.6845, 121.031)
  line L49 (-15.6845, 121.031) -> (-2.9845, 121.031)
  line L50 (-2.9845, 121.031) -> (-2.9845, 127)
  line L51 (2.9845, 228.6) -> (2.9845, 203.2) construction
  line L52 (-2.9845, 228.6) -> (-2.9845, 203.2) construction
  line L53 (2.9845, 203.2) -> (15.6845, 203.2)
  line L54 (15.6845, 203.2) -> (15.6845, 197.231)
  line L55 (15.6845, 197.231) -> (2.9845, 197.231)
  line L56 (2.9845, 197.231) -> (2.9845, 203.2)
  line L57 (-2.9845, 203.2) -> (-15.6845, 203.2)
  line L58 (-15.6845, 203.2) -> (-15.6845, 197.231)
  line L59 (-15.6845, 197.231) -> (-2.9845, 197.231)
  line L60 (-2.9845, 197.231) -> (-2.9845, 203.2)
  line L61 (2.9845, 177.8) -> (2.9845, 152.4) construction
  line L62 (-2.9845, 177.8) -> (-2.9845, 152.4) construction
  line L63 (2.9845, 152.4) -> (15.6845, 152.4)
  line L64 (15.6845, 152.4) -> (15.6845, 146.431)
  line L65 (15.6845, 146.431) -> (2.9845, 146.431)
  line L66 (2.9845, 146.431) -> (2.9845, 152.4)
  line L67 (-2.9845, 152.4) -> (-15.6845, 152.4)
  line L68 (-15.6845, 152.4) -> (-15.6845, 146.431)
  line L69 (-15.6845, 146.431) -> (-2.9845, 146.431)
  line L70 (-2.9845, 146.431) -> (-2.9845, 152.4)
  line L71 (2.9845, 127) -> (2.9845, 101.6) construction
  line L72 (-2.9845, 127) -> (-2.9845, 101.6) construction
  line L73 (2.9845, 101.6) -> (15.6845, 101.6)
  line L74 (15.6845, 101.6) -> (15.6845, 95.631)
  line L75 (15.6845, 95.631) -> (2.9845, 95.631)
  line L76 (2.9845, 95.631) -> (2.9845, 101.6)
  line L77 (-2.9845, 101.6) -> (-15.6845, 101.6)
  line L78 (-15.6845, 101.6) -> (-15.6845, 95.631)
  line L79 (-15.6845, 95.631) -> (-2.9845, 95.631)
  line L80 (-2.9845, 95.631) -> (-2.9845, 101.6)
  dimension "d114" = 76.2
  dimension "d115" = 2.9845
  dimension "d116" = 2.9845
  dimension "d117" = 12.7
  dimension "d118" = 5.969
  dimension "d119" = 12.7
  dimension "d120" = 5.969
  dimension "d121" = 50.8
  dimension "d122" = 50.8
  dimension "d123" = 12.7
  dimension "d124" = 5.969
  dimension "d125" = 12.7
  dimension "d126" = 5.969
  dimension "d127" = 50.8
  dimension "d128" = 50.8
  dimension "d129" = 12.7
  dimension "d130" = 5.969
  dimension "d131" = 12.7
  dimension "d132" = 5.969
  dimension "d133" = 25.4
  dimension "d134" = 25.4
  dimension "d135" = 12.7
  dimension "d136" = 5.969
  dimension "d137" = 12.7
  dimension "d138" = 5.969
  dimension "d139" = 25.4
  dimension "d140" = 25.4
  dimension "d141" = 12.7
  dimension "d142" = 5.969
  dimension "d143" = 12.7
  dimension "d144" = 5.969
  dimension "d147" = 25.4
  dimension "d148" = 25.4
  dimension "d149" = 12.7
  dimension "d150" = 5.969
  dimension "d151" = 12.7
  dimension "d152" = 5.969
  constraint midpoint L0 L20.start
  constraint perpendicular L0 L20
  constraint perpendicular L20 L21
  constraint perpendicular L20 L22
  constraint horizontal L23
  constraint vertical L24
  constraint horizontal L25
  constraint vertical L26
  constraint horizontal L27
  constraint vertical L28
  constraint horizontal L29
  constraint vertical L30
  constraint perpendicular L25 L31
  constraint perpendicular L22 L32
  constraint horizontal L33
  constraint vertical L34
  constraint horizontal L35
  constraint vertical L36
  constraint horizontal L37
  constraint vertical L38
  constraint horizontal L39
  constraint vertical L40
  constraint perpendicular L35 L41
  constraint perpendicular L39 L42
  constraint horizontal L43
  constraint vertical L44
  constraint horizontal L45
  constraint vertical L46
  constraint horizontal L47
  constraint vertical L48
  constraint horizontal L49
  constraint vertical L50
  constraint perpendicular L25 L51
  constraint vertical L52
  constraint horizontal L53
  constraint vertical L54
  constraint horizontal L55
  constraint vertical L56
  constraint horizontal L57
  constraint vertical L58
  constraint horizontal L59
  constraint vertical L60
  constraint perpendicular L35 L61
  constraint perpendicular L39 L62
  constraint horizontal L63
  constraint vertical L64
  constraint horizontal L65
  constraint vertical L66
  constraint horizontal L67
  constraint vertical L68
  constraint horizontal L69
  constraint vertical L70
  constraint perpendicular L45 L71
  constraint perpendicular L47 L72
  constraint horizontal L73
  constraint vertical L74
  constraint horizontal L75
  constraint vertical L76
  constraint horizontal L77
  constraint vertical L78
  constraint horizontal L79
  constraint vertical L80
  measures "d114" distance of L20.start L20.end
  measures "d115" distance of L20.end L21.end
  measures "d116" distance of L20.end L22.end
  measures "d117" distance of L21.end L23.end
  measures "d118" distance of L21.end L25.end
  measures "d119" distance of L22.end L27.end
  measures "d120" distance of L22.end L29.end
  measures "d121" distance of L21.end L31.end
  measures "d122" distance of L22.end L32.end
  measures "d123" distance of L31.end L33.end
  measures "d124" distance of L31.end L35.end
  measures "d125" distance of L32.end L37.end
  measures "d126" distance of L32.end L39.end
  measures "d127" distance of L31.end L41.end
  measures "d128" distance of L32.end L42.end
  measures "d129" distance of L41.end L43.end
  measures "d130" distance of L41.end L45.end
  measures "d131" distance of L42.end L47.end
  measures "d132" distance of L42.end L49.end
  measures "d133" distance of L21.end L51.end
  measures "d134" distance of L22.end L52.end
  measures "d135" distance of L51.end L53.end
  measures "d136" distance of L51.end L55.end
  measures "d137" distance of L52.end L57.end
  measures "d138" distance of L52.end L59.end
  measures "d139" distance of L31.end L61.end
  measures "d140" distance of L32.end L62.end
  measures "d141" distance of L61.end L63.end
  measures "d142" distance of L61.end L65.end
  measures "d143" distance of L62.end L67.end
  measures "d144" distance of L62.end L69.end
  measures "d147" distance of L41.end L71.end
  measures "d148" distance of L42.end L72.end
  measures "d149" distance of L71.end L73.end
  measures "d150" distance of L71.end L75.end
  measures "d151" distance of L72.end L77.end
  measures "d152" distance of L72.end L79.end